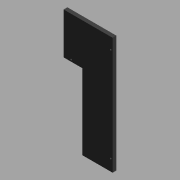
# Autodesk Inventor part: box_front_right
Saved by Autodesk Inventor 2019 (Build 230136000, 136)
## iProperties
Part Number: box_front_right
Material: Generic
Document SubType Name: Modeling
Designer: Javi
Appearance: Default
Author: Javi
Autodesk Inventor part; units mm, degrees
ref_plane "YZ Plane" through (0, 0, 0) normal (1, 0, 0) x (0, 1, 0)
ref_plane "XZ Plane" through (0, 0, 0) normal (0, 1, 0) x (-1, 0, 0)
ref_plane "XY Plane" through (0, 0, 0) normal (0, 0, 1) x (1, 0, 0)
sketch "Sketch3" plane through (0, 0, 0) normal (0, 1, 0) x (-1, 0, 0)
  line L0 (0, 0) -> (80, 0)
  line L1 (62.6378, -10) -> (0, -10)
  line L2 (0, -10) -> (0, 0)
  arc A0 (80, 0) -> (62.6378, -10) centre (130, -106.8831) ccw
  point P0 (34, -10)
  dimension "d20" = 118
  dimension "d22" = 10
  dimension "d23" = 50
  dimension "d24" = 80
  constraints: 6 end point, 2 point on circle, 1 centre point, 1 horizontal, 1 parallel, 1 point on line, 1 vertical
  measures "d20" radius of A0
  measures "d22" distance between parallel lines of L0 L1
  measures "d23" horizontal distance of L0.end A0.centre
  measures "d24" distance of L0.start L0.end
extrude "Extrusion3" add sketch "Sketch3" along normal blind 200
sketch "Sketch6" plane through (0, 200, 0) normal (0, 1, 0) x (1, 0, 0)
  line L0 (-80, 0) -> (0, 0) projected
  line L1 (0, 0) -> (-130, 0)
  line L2 (-130, 0) -> (-130, 10)
  line L3 (-130, 10) -> (0, 10)
  line L4 (0, 10) -> (0, 0)
  dimension "d42" = 130
  dimension "d43" = 10
  constraints: 8 end point, 2 parallel, 1 horizontal, 1 perpendicular
  measures "d42" distance of L2.end L3.end
  measures "d43" distance of L1.end L2.end
sketch "Sketch5" plane through (0, 0, 0) normal (0, -1, 0) x (1, 0, 0)
  circle A0 centre (-30, -5) radius 2
  line L0 (0, -10) -> (0, 0) projected
  line L1 (0, 0) -> (-80, 0) projected
  dimension "d37" = 4
  dimension "d38" = 30
  dimension "d39" = 5
  constraints: 1 centre point
  measures "d37" diameter of A0
  measures "d38" distance from line of L0 A0.centre
  measures "d39" distance from line of L1 A0.centre
extrude "Extrusion5" cut sketch "Sketch5" against normal blind 20
sketch "Sketch4" plane through (-80, 0, 0) normal (0, 0, 1) x (1, 0, 0)
  circle A0 centre (75, 30) radius 2
  line L0 (80, 0) -> (80, 200) projected
  line L1 (80, 0) -> (0, 0) projected
  circle A1 centre (75, 280) radius 2
  dimension "d25" = 4
  dimension "d26" = 5
  dimension "d27" = 30
  dimension "d30" = 250
  constraints: 2 centre point, 1 vertical, 2 other
  measures "d25" diameter of A0
  measures "d26" distance from line of L0 A0.centre
  measures "d27" distance from line of L1 A0.centre
  measures "d30" distance of A0.centre A1.centre
extrude "Extrusion6" add sketch "Sketch6" along normal blind 110
extrude "Extrusion7" cut sketch "Sketch4" against normal through all
sketch "Sketch7" plane through (-80, 0, 0) normal (0, 0, 1) x (1, 0, 0)
  circle A0 centre (-30, 205) radius 2
  line L0 (0, 200) -> (-50, 200) projected
  line L1 (-50, 200) -> (-50, 310) projected
  point P0 (80, 0)
  dimension "d48" = 4
  dimension "d49" = 5
  dimension "d50" = 20
  constraints: 1 centre point
  measures "d48" diameter of A0
  measures "d49" distance from line of L0 A0.centre
  measures "d50" distance from line of L1 A0.centre
extrude "Extrusion8" cut sketch "Sketch7" against normal through all
equation "\"d48\" = screws"
equation "\"screws\" = 4"
body "Solid3"
